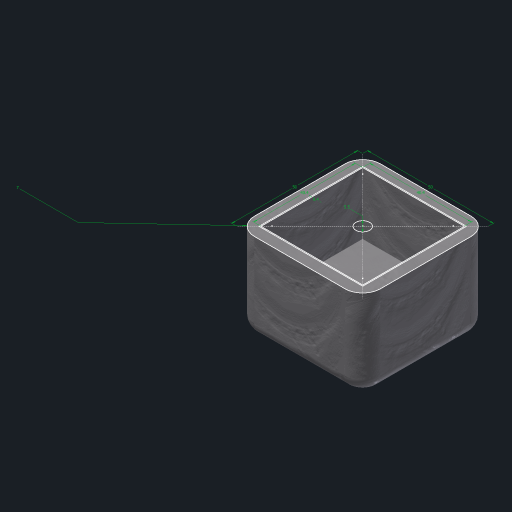
# Autodesk Inventor part: PATA_PLASTICO
Saved by Autodesk Inventor 2024.3 (Build 283343000, 343)
## iProperties
Created: 2024-07-16
Part Number: PATA_PLASTICO
Material: Steel, Mild, Welded
Document SubType Name: Modeling
Designer: Niler
Density: 7.85 g/cm^3
Appearance: Weld - Steel Mild
Author: Niler
Autodesk Inventor part; units mm, degrees
ref_plane "YZ Plane" through (0, 0, 0) normal (1, 0, 0) x (0, 1, 0)
ref_plane "XZ Plane" through (0, 0, 0) normal (0, 1, 0) x (-1, 0, 0)
ref_plane "XY Plane" through (0, 0, 0) normal (0, 0, 1) x (1, 0, 0)
sketch "Sketch1" plane through (0, 0, 0) normal (0, 1, 0) x (-1, 0, 0)
  line L0 (-18, 25) -> (18, 25)
  line L1 (25, 18) -> (25, -18)
  line L2 (18, -25) -> (-18, -25)
  line L3 (-25, -18) -> (-25, 18)
  line L4 (-25, 25) -> (25, -25) construction
  line L5 (25, 25) -> (-25, -25) construction
  circle A0 centre (0, 0) radius 2.75
  arc A1 (25, 18) -> (18, 25) centre (18, 18) ccw
  arc A2 (18, -25) -> (25, -18) centre (18, -18) ccw
  arc A3 (-25, -18) -> (-18, -25) centre (-18, -18) ccw
  arc A4 (-18, 25) -> (-25, 18) centre (-18, 18) ccw
  line L6 (-20.2, 20.2) -> (20.2, 20.2)
  line L7 (20.2, 20.2) -> (20.2, -20.2)
  line L8 (20.2, -20.2) -> (-20.2, -20.2)
  line L9 (-20.2, -20.2) -> (-20.2, 20.2)
  line L10 (-20.2, 20.2) -> (20.2, -20.2) construction
  line L11 (20.2, 20.2) -> (-20.2, -20.2) construction
  line L12 (20.6, -20.6) -> (20.6, 20.6)
  line L13 (20.6, 20.6) -> (-20.6, 20.6)
  line L14 (-20.6, 20.6) -> (-20.6, -20.6)
  line L15 (-20.6, -20.6) -> (20.6, -20.6)
  dimension "d0" = 50
  dimension "d1" = 50
  dimension "d2" = 5.5
  dimension "d3" = 7
  dimension "d4" = 40.4
  dimension "d5" = 40.4
  dimension "d8" = 0.4
  constraints: 32 end point, 8 point on circle, 8 point on line, 8 tangent, 6 parallel, 5 centre point, 4 midpoint, 3 equal radius, 3 perpendicular, 2 horizontal, 1 coincident, 3 other
  measures "d0" distance of L4.end L5.end
  measures "d1" distance of L5.start L4.end
  measures "d2" diameter of A0
  measures "d3" radius of A1
  measures "d4" distance of L7.end L8.end
  measures "d5" distance of L6.end L7.end
  measures "d8" distance between parallel lines of L7 L12
extrude "Extrusion1" add sketch "Sketch1" against normal blind 35 contours L0 A1 L1 A2 L2 A3 L3 A4 | A0 | L6 L7 L8 L9 | L15 L14 L13 L12
fillet "Fillet1" radius 5 8 edges at (0, -35, 25) (-22.9497, -35, 22.9497) (-25, -35, 0) (-22.9497, -35, -22.9497) (0, -35, -25) (22.9497, -35, -22.9497) (25, -35, 0) (22.9497, -35, 22.9497)
extrude "Extrusion2" cut sketch "Sketch1" against normal blind 25 contours A0 | L6 L7 L8 L9 | L15 L14 L13 L12
sketch "Sketch2" plane through (0, -35, 0) normal (0, -1, 0) x (1, 0, 0)
  circle A0 centre (0, 0) radius 2.75 projected
  line L0 (-10.5, 12.5) -> (10.5, 12.5) projected
  arc A1 (-10.5, 12.5) -> (-12.5, 10.5) centre (-10.5, 10.5) ccw projected
  line L1 (-12.5, -10.5) -> (-12.5, 10.5) projected
  arc A2 (-12.5, -10.5) -> (-10.5, -12.5) centre (-10.5, -10.5) ccw projected
  line L2 (10.5, -12.5) -> (-10.5, -12.5) projected
  arc A3 (10.5, -12.5) -> (12.5, -10.5) centre (10.5, -10.5) ccw projected
  line L3 (12.5, 10.5) -> (12.5, -10.5) projected
  arc A4 (12.5, 10.5) -> (10.5, 12.5) centre (10.5, 10.5) ccw projected
  circle A5 centre (0, 0) radius 5
  dimension "d12" = 10
  constraints: 1 centre point, 1 coincident
  measures "d12" diameter of A5
body "Solid1"
